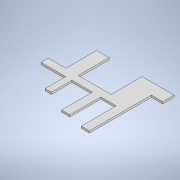
# Autodesk Inventor part: medium_obstacle
Saved by Autodesk Inventor 2020.2 (Build 242310000, 310)
## iProperties
Created: 2021-03-12
Part Number: medium_obstacle
Material: Generic
Document SubType Name: Modeling
Designer: Tarsoly
Density: 1 g/cm^3
Appearance: Default
Author: Tarsoly
Autodesk Inventor part; units mm, degrees
ref_plane "YZ Plane" through (0, 0, 0) normal (1, 0, 0) x (0, 1, 0)
ref_plane "XZ Plane" through (0, 0, 0) normal (0, 1, 0) x (-1, 0, 0)
ref_plane "XY Plane" through (0, 0, 0) normal (0, 0, 1) x (1, 0, 0)
sketch "Sketch1" plane through (0, 0, 0) normal (0, 1, 0) x (-1, 0, 0)
  line L0 (2500, 2500) -> (-2500, 2500)
  line L1 (-2500, 2500) -> (-2500, -2500)
  line L2 (-2500, -2500) -> (2500, -2500)
  line L3 (2500, -2500) -> (2500, 2500)
  line L4 (2500, 2500) -> (-2500, -2500) construction
  line L5 (-2500, 2500) -> (2500, -2500) construction
  line L6 (2500, 350) -> (1300, 350)
  line L7 (1300, 350) -> (1300, 1350)
  line L8 (1300, 1350) -> (1000, 1350)
  line L9 (1000, 1350) -> (1000, 350)
  line L10 (1000, 350) -> (0, 350)
  line L11 (-400, 350) -> (-1150, 350)
  line L12 (-1150, 350) -> (-1150, 2050)
  line L13 (-1150, 2050) -> (-1550, 2050)
  line L14 (-1550, 2050) -> (-1550, -950)
  line L15 (-1550, -950) -> (-2100, -950)
  line L16 (-2100, -950) -> (-2100, -1500)
  line L17 (-2100, -1500) -> (-550, -1500)
  line L18 (-550, -1500) -> (-550, 0)
  line L19 (-550, 0) -> (1050, 0)
  line L20 (1050, 0) -> (1050, -1500)
  line L21 (1050, -1500) -> (1650, -1500)
  line L22 (1650, -1500) -> (1650, 0)
  line L23 (1650, 0) -> (2500, 0)
  line L24 (0, 350) -> (0, 1850)
  line L25 (0, 1850) -> (-400, 1850)
  line L26 (-400, 1850) -> (-400, 350)
  point P0 (0, 0)
  dimension "d0" = 5000
  dimension "d1" = 5000
  dimension "d2" = 1200
  dimension "d3" = 300
  dimension "d4" = 1000
  dimension "d5" = 2500
  dimension "d6" = 350
  dimension "d7" = 850
  dimension "d8" = 600
  dimension "d10" = 1500
  dimension "d12" = 400
  dimension "d13" = 1000
  dimension "d14" = 750
  dimension "d15" = 400
  dimension "d16" = 1700
  dimension "d17" = 400
  dimension "d18" = 3000
  dimension "d19" = 1000
  dimension "d20" = 1600
  constraints: 54 end point, 16 perpendicular, 5 point on line, 3 midpoint, 2 collinear, 2 horizontal, 2 parallel, 1 vertical
  measures "d0" distance of L2.end L1.end
  measures "d1" distance of L1.end L0.end
  measures "d2" distance of L6.start L6.end
  measures "d3" distance of L7.end L8.end
  measures "d4" distance of L6.end L7.end
  measures "d5" distance between parallel lines of L2 L23
  measures "d6" distance between parallel lines of L6 L23
  measures "d7" distance of L22.end L23.end
  measures "d8" distance of L20.end L21.end
  measures "d10" distance of L10.end L24.end
  measures "d12" distance of L24.end L25.end
  measures "d13" distance of L9.end L10.end
  measures "d14" distance of L11.start L11.end
  measures "d15" distance of L12.end L13.end
  measures "d16" distance of L11.end L12.end
  measures "d17" distance between parallel lines of L1 L16
  measures "d18" distance of L13.end L14.end
  measures "d19" distance between parallel lines of L2 L17
  measures "d20" distance between parallel lines of L18 L20
extrude "Extrusion1" add sketch "Sketch1" along normal blind 100 contours L3 L23 L22 L21 L20 L19 L18 L17 L16 L15 L14 L13 L12 L11 L26 L25 L24 L10 L9 L8 L7 L6
body "Solid1"
